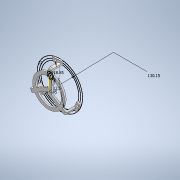
# Autodesk Inventor part: Return_Spool_Mount_2
Saved by Autodesk Inventor 2022 (Build 260153070, 153G)
## iProperties
Created: 2022-03-05
Part Number: Return_Spool_Mount_2
Material: Generic
Document SubType Name: Modeling
Designer: a laptop
Density: 1 g/cm^3
Appearance: Default
Author: a laptop
Autodesk Inventor part; units mm, degrees
ref_plane "YZ Plane" through (0, 0, 0) normal (1, 0, 0) x (0, 1, 0)
ref_plane "XZ Plane" through (0, 0, 0) normal (0, 1, 0) x (-1, 0, 0)
ref_plane "XY Plane" through (0, 0, 0) normal (0, 0, 1) x (1, 0, 0)
sketch "Sketch1" plane through (0, 0, 0) normal (0, 0, 1) x (1, 0, 0)
  circle A0 centre (0, 0) radius 59.425
  circle A1 centre (0, 0) radius 71.425
  line L0 (0, 0) -> (0, 59.425) construction
  line L1 (0, 71.425) -> (0, 59.425) construction
  circle A2 centre (0, 0) radius 65.075
  dimension "d0" = 118.85
  dimension "d2" = 12
  dimension "d12" = 130.15
  constraints: 4 end point, 2 coincident, 2 vertical alignment, 1 centre point, 1 collinear, 1 point on line, 1 vertical, 5 other
  measures "d12" diameter of A2
sketch "Sketch2" plane through (0, 0, 0) normal (1, 0, 0) x (0, 1, 0)
  line L0 (59.425, 0) -> (59.425, 25)
  line L1 (54.425, 30) -> (0, 30)
  line L2 (59.425, 35) -> (0, 35)
  line L3 (0, 35) -> (0, 30)
  line L4 (71.425, 0) -> (71.425, 5)
  line L5 (71.425, 5) -> (64.425, 5)
  line L6 (64.425, 5) -> (64.425, 30)
  arc A0 (64.425, 30) -> (59.425, 35) centre (59.425, 30) ccw
  arc A1 (59.425, 25) -> (54.425, 30) centre (54.425, 25) ccw
  line L7 (71.425, 0) -> (59.425, 0)
  point P0 (0, 0)
  dimension "d3" = 5
  dimension "d5" = 30
  dimension "d6" = 5
  dimension "d7" = 5
  dimension "d8" = 5
  constraints: 16 end point, 4 perpendicular, 4 point on circle, 4 tangent, 2 centre point, 2 point on line, 2 vertical, 1 equal radius, 1 horizontal, 1 vertical alignment
  measures "d3" distance between parallel lines of L2 L1
  measures "d5" distance of point (59.425, 30) L0.start
  measures "d6" distance between parallel lines of L0 L6
  measures "d7" radius of A0
  measures "d8" distance from line of L4.start L5
extrude "Extrusion2" add sketch "Sketch2" along normal blind 10
sketch "Sketch5" plane through (0, 0, 0) normal (-1, 0, 0) x (0, 0, 1)
  line L0 (5, 71.425) -> (0, 71.425)
  line L1 (0, 71.425) -> (0, 59.425)
  line L2 (0, 59.425) -> (5, 59.425)
  line L3 (5, 59.425) -> (5, 71.425)
  line L4 (-7, 0) -> (42, 0) projected
  point P0 (0, 0)
  constraints: 8 end point, 2 coincident, 2 parallel, 1 horizontal, 1 perpendicular
revolve "Revolution1" add sketch "Sketch5" angle 15 about axis through (0, 0, -10) along (0, 0, 1)
sketch "Sketch6" plane through (0, 64.425, 5) normal (0, 0, 1) x (1, 0, 0)
  circle A0 centre (0, -64.425) radius 65.075 construction
  circle A1 centre (-8.494, 0.0933) radius 4
  line L0 (-8.494, 0.0933) -> (0, 7) construction
  line L1 (-18.4862, 4.5663) -> (-8.494, 0.0933) construction
  dimension "d17" = 8
  constraints: 4 end point, 1 centre point, 1 equal length, 2 other
  measures "d17" diameter of A1
extrude "Extrusion3" cut sketch "Sketch6" against normal blind 10
pattern_circular "Circular Pattern1" count 3 over 360 about axis through (0, 0, -10) along (0, 0, 1) of "Extrusion2", "Revolution1", "Extrusion3"
sketch "Sketch7" plane through (0, 59.425, 35) normal (0, 0, 1) x (1, 0, 0)
  circle A0 centre (0, -59.425) radius 50
  circle A1 centre (0, -59.425) radius 40
  circle A2 centre (0, -59.425) radius 65.075 projected
  circle A3 centre (0, -59.425) radius 10
  point P0 (-5, -50.7647)
  dimension "d23" = 100
  dimension "d24" = 80
  constraints: 2 centre point, 1 coincident, 1 concentric, 4 other
  measures "d23" diameter of A0
  measures "d24" diameter of A1
extrude "Extrusion4" add sketch "Sketch7" against normal blind 5 contours A0 | A3
sketch "Sketch8" plane through (0, 59.425, 35) normal (0, 0, 1) x (1, 0, 0)
  circle A0 centre (5, -14.425) radius 6.25
  line L0 (0, -19.425) -> (0, -49.425) projected
  circle A1 centre (5, -14.425) radius 12.25
  circle A2 centre (-2.7942, -9.925) radius 1.5
  circle A3 centre (5, -23.425) radius 1.5
  circle A4 centre (12.7942, -9.925) radius 1.5
  circle A5 centre (5, -14.425) radius 9 construction
  line L1 (5, -23.425) -> (-2.7942, -9.925) construction
  line L2 (12.7942, -9.925) -> (-2.7942, -9.925) construction
  line L3 (5, -23.425) -> (12.7942, -9.925) construction
  point P0 (0, -59.425)
  dimension "d27" = 12.5
  dimension "d28" = 5
  dimension "d29" = 45
  dimension "d32" = 6
  dimension "d35" = 3
  dimension "d36" = 3
  dimension "d37" = 3
  dimension "d38" = 18
  constraints: 6 centre point, 6 end point, 3 point on circle, 2 equal length, 1 coincident, 1 concentric, 1 horizontal
  measures "d27" diameter of A0
  measures "d28" distance from line of L0 A0.centre
  measures "d29" vertical distance of point (0, -59.425) A0.centre
  measures "d32" radial gap between concentric circles of A1 A0
  measures "d35" diameter of A2
  measures "d36" diameter of A3
  measures "d37" diameter of A4
  measures "d38" diameter of A5
extrude "Extrusion6" add sketch "Sketch8" against normal blind 5 contours A1 | A2 | A3 | A4
extrude "Extrusion5" cut sketch "Sketch8" against normal blind 5 contours A0 | A2 | A3 | A4
body "Solid2"
